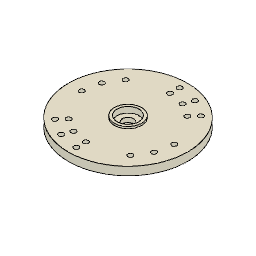
Disc Servo Attachment (Autodesk Fusion 360 design; units mm, degrees)
Autodesk Fusion 360 part; units mm, degrees
sketch "Sketch1" plane through (0, 0, 0) normal (0, 1, 0) x (1, 0, 0)
  circle A0 centre (0, 0) radius 3.4163
  circle A1 centre (0, 0) radius 2.3241
  dimension "d1" = 6.8326
  dimension "d2" = 4.6482
  constraint coincident A0.centre A1.centre
  constraint concentric A0 A1
  measures "d1" diameter of A0
  measures "d2" diameter of A1
extrude "Extrude1" add sketch "Sketch1" along normal blind 2.3368 makes body 1
sketch "Sketch2" plane through (0, 2.3368, 0) normal (0, 1, 0) x (-1, 0, 0)
  circle A0 centre (0, 0) radius 2.3241
  circle A1 centre (0, 0) radius 3.4163
  circle A2 centre (0, 0) radius 11.8872
  circle A3 centre (0, 0) radius 1.1303
  dimension "d5" = 23.7744
  dimension "d6" = 2.2606
  constraint coincident A0.centre A1.centre
  constraint concentric A2 A3
  measures "d5" diameter of A2
  measures "d6" diameter of A3
extrude "Extrude2" add sketch "Sketch2" along normal blind 1.651 separate body contours A0 | A1 | A2 makes body 2
sketch "Sketch3" plane through (0, 3.9878, 0) normal (0, 1, 0) x (-1, 0, 0)
  circle A0 centre (0, 0) radius 1.1303
  circle A1 centre (0, 0) radius 11.8872
  circle A2 centre (0, 0) radius 2.7178
  circle A3 centre (0, 0) radius 2.1844
  dimension "d9" = 5.4356
  dimension "d10" = 4.3688
  constraint concentric A0 A2
  constraint coincident A0.centre A1.centre
  measures "d9" diameter of A2
  measures "d10" diameter of A3
extrude "Extrude3" add sketch "Sketch3" along normal blind 0.381 contours A2 bodies 2
sketch "Sketch4" plane through (0, 3.9878, 0) normal (0, 1, 0) x (-1, 0, 0)
  circle A0 centre (0, 0) radius 11.8872
  circle A1 centre (0, 0) radius 2.7178
  circle A2 centre (0, 0) radius 10.2872 construction
  circle A3 centre (0, 0) radius 9.2202 construction
  circle A4 centre (0, 0) radius 8.382 construction
  line L0 (0, 2.7178) -> (0, -10.795) construction
  circle A5 centre (-0.0124, -10.2872) radius 0.508
  circle A6 centre (0, -8.382) radius 0.508
  circle A7 centre (0, 0) radius 11.8872 construction
  line L1 (0, -10.795) -> (0, -11.8872) construction
  line L2 (0, -11.8872) -> (0, -8.89) construction
  circle A8 centre (-3.0695, -7.7998) radius 0.508
  circle A9 centre (-3.7556, -9.5771) radius 0.508
  circle A10 centre (-5.6936, -6.1515) radius 0.508
  circle A11 centre (-6.9837, -7.5534) radius 0.508
  line L3 (0.4991, -8.4767) -> (-3.5686, -7.7051) construction
  line L4 (0.4867, -10.3818) -> (-4.2547, -9.4824) construction
  line L5 (-2.6393, -8.07) -> (-6.1237, -5.8813) construction
  line L6 (-3.3252, -9.8469) -> (-7.4141, -7.2835) construction
  line L7 (0, 0) -> (-11.8872, 0) construction
  circle A12 centre (-9.2202, 0) radius 0.508
  line L8 (-11.8872, 0) -> (-9.7282, 0) construction
  circle A13 centre (-8.5826, 3.3692) radius 0.508
  circle A14 centre (-6.7579, 6.2724) radius 0.508
  line L9 (-9.3147, -0.4991) -> (-8.4881, 3.8683) construction
  line L10 (-8.8529, 2.9391) -> (-6.4876, 6.7025) construction
  circle A15 centre (0.0124, 10.2872) radius 0.508
  circle A16 centre (0, 8.382) radius 0.508
  circle A17 centre (3.7556, 9.5771) radius 0.508
  circle A18 centre (3.0695, 7.7998) radius 0.508
  circle A19 centre (6.9837, 7.5534) radius 0.508
  circle A20 centre (5.6936, 6.1515) radius 0.508
  circle A21 centre (9.2202, 0) radius 0.508
  circle A22 centre (8.5826, -3.3692) radius 0.508
  circle A23 centre (6.7579, -6.2724) radius 0.508
  dimension "d13" = 1.016
  dimension "d14" = 1.016
  dimension "d16" = 1.0922
  dimension "d17" = 2.9972
  dimension "d18" = 1.016
  dimension "d19" = 1.016
  dimension "d20" = 1.016
  dimension "d21" = 1.016
  dimension "d22" = 4.1402
  dimension "d23" = 4.826
  dimension "d24" = 4.1148
  dimension "d25" = 4.826
  dimension "d26" = 1.016
  dimension "d27" = 2.159
  dimension "d28" = 1.016
  dimension "d29" = 1.016
  dimension "d30" = 4.445
  dimension "d31" = 4.445
  dimension "d32" = 1.016
  dimension "d33" = 1.016
  dimension "d34" = 1.016
  dimension "d35" = 1.016
  dimension "d36" = 1.016
  dimension "d37" = 1.016
  dimension "d38" = 1.016
  dimension "d39" = 1.016
  dimension "d40" = 1.016
  constraint concentric A0 A2
  constraint concentric A0 A3
  constraint coincident A0.centre A1.centre
  constraint vertical L0
  constraint coincident A4 A6.centre
  constraint coincident L0 A6.centre
  constraint coincident A1 L0.start
  constraint concentric A4 A7
  constraint equal A0 A7
  constraint coincident A5 L0.end
  constraint coincident A7 L1.end
  constraint parallel L0 L1
  constraint coincident L0 L2.end
  constraint coincident A6 L2.end
  constraint coincident A2 A5.centre
  constraint coincident A4 A8.centre
  constraint coincident A2 A9.centre
  constraint coincident A4 A10.centre
  constraint coincident A2 A11.centre
  constraint coincident A6 L3.start
  constraint coincident A8 L3.end
  constraint coincident A5 L4.start
  constraint coincident A9 L4.end
  constraint parallel L3 L4
  constraint coincident A6.centre L3
  constraint coincident A8.centre L3
  constraint coincident A5.centre L4
  constraint coincident A9.centre L4
  constraint coincident A8 L5.start
  constraint coincident A10 L5.end
  constraint coincident A9 L6.start
  constraint coincident A11 L6.end
  constraint coincident A8.centre L5
  constraint coincident A10.centre L5
  constraint coincident A9.centre L6
  constraint coincident A11.centre L6
  constraint coincident A7 L7.end
  constraint perpendicular L0 L7
  constraint coincident A3 A12.centre
  constraint coincident L7 A12.centre
  constraint coincident A12 L8.end
  constraint coincident L7 L8.end
  constraint coincident A3 A13.centre
  constraint coincident A3 A14.centre
  constraint coincident A12 L9.start
  constraint coincident A13 L9.end
  constraint coincident A13 L10.start
  constraint coincident A14 L10.end
  constraint coincident A12.centre L9
  constraint coincident A13.centre L9
  constraint coincident A13.centre L10
  constraint coincident A14.centre L10
  constraint coincident A0.centre L0
  measures "d13" diameter of A5
  measures "d14" diameter of A6
  measures "d16" distance of L0.end L1.end
  measures "d17" distance of L1.end L2.end
  measures "d18" diameter of A8
  measures "d19" diameter of A9
  measures "d20" diameter of A10
  measures "d21" diameter of A11
  measures "d22" distance of L3.start L3.end
  measures "d23" distance of L4.start L4.end
  measures "d24" distance of L5.start L5.end
  measures "d25" distance of L6.start L6.end
  measures "d26" diameter of A12
  measures "d27" distance of L7.end L8.end
  measures "d28" diameter of A13
  measures "d29" diameter of A14
  measures "d30" distance of L9.start L9.end
  measures "d31" distance of L10.start L10.end
  measures "d32" diameter of A15
  measures "d33" diameter of A16
  measures "d34" diameter of A18
  measures "d35" diameter of A17
  measures "d36" diameter of A20
  measures "d37" diameter of A19
  measures "d38" diameter of A21
  measures "d39" diameter of A22
  measures "d40" diameter of A23
hole "Hole1" at (0.0124, 3.9878, -10.2872) at (0, 3.9878, -8.382) at (3.7556, 3.9878, -9.5771) at (3.0695, 3.9878, -7.7998) at (6.9837, 3.9878, -7.5534) at (5.6936, 3.9878, -6.1515) at (9.2202, 3.9878, 0) at (8.5826, 3.9878, 3.3692) at (6.7579, 3.9878, 6.2724) at (-0.0124, 3.9878, 10.2872) at (0, 3.9878, 8.382) at (-3.0695, 3.9878, 7.7998) at (-3.7556, 3.9878, 9.5771) at (-6.9837, 3.9878, 7.5534) at (-5.6936, 3.9878, 6.1515) at (-9.2202, 3.9878, 0) at (-8.5826, 3.9878, -3.3692) at (-6.7579, 3.9878, -6.2724) direction (0, -1, 0) diameter 1 end through all bodies 2
extrude "Extrude4" cut 1 faces at (-1.8207, 3.9878, -0.1647) along direction (0, -1, 0) blind 1.143 from surface at -0.381 on bodies 2 bodies 2
